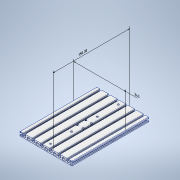
# Autodesk Inventor part: T_20240
Saved by Autodesk Inventor 2021 (Build 250183000, 183)
## iProperties
Created: 2022-05-22
Part Number: T_20240
Material: Aluminio 6061
Document SubType Name: Modeling
Designer: 79449
Density: 2.7 g/cm^3
Appearance: Aluminio - Plano
Author: 79449
Autodesk Inventor part; units mm, degrees
ref_plane "YZ Plane" through (0, 0, 0) normal (1, 0, 0) x (0, 1, 0)
ref_plane "XZ Plane" through (0, 0, 0) normal (0, 1, 0) x (-1, 0, 0)
ref_plane "XY Plane" through (0, 0, 0) normal (0, 0, 1) x (1, 0, 0)
sketch "Boceto1" plane through (0, 0, 0) normal (0, 0, 1) x (1, 0, 0)
  line L0 (-120, 0) -> (120, 0)
  line L1 (-120, 0) -> (-120, 20) construction
  line L2 (-120, 20) -> (120, 20) construction
  line L3 (120, 20) -> (120, 0) construction
  line L4 (-120, 14.15) -> (-117.15, 14.15)
  line L5 (-120, 5.85) -> (-117.15, 5.85)
  line L6 (-117.15, 2.85) -> (-110.15, 2.85)
  line L7 (-117.15, 5.85) -> (-117.15, 2.85)
  line L8 (-117.15, 14.15) -> (-117.15, 17.15)
  line L9 (-117.15, 17.15) -> (-110.15, 17.15)
  line L10 (-120, 5.85) -> (-120, 0)
  line L11 (-120, 14.15) -> (-120, 20)
  line L12 (-120, 20) -> (-104, 20)
  line L13 (-104, 20) -> (-104, 16)
  line L14 (-104, 16) -> (-107, 16)
  line L15 (-107, 16) -> (-107, 8.85)
  line L16 (-107, 8.85) -> (-104, 8.85)
  line L17 (-104, 8.85) -> (-104, 6)
  line L18 (-104, 6) -> (-95.7, 6)
  line L19 (-95.7, 6) -> (-95.7, 8.85)
  line L20 (-95.7, 8.85) -> (-92.7, 8.85)
  line L21 (-92.7, 8.85) -> (-92.7, 16)
  line L22 (-92.7, 16) -> (-95.7, 16)
  line L23 (-95.7, 16) -> (-95.7, 20)
  line L24 (-95.7, 20) -> (-79.9, 20)
  line L25 (-84.05, 14) -> (-75.75, 14)
  line L26 (-79.9, 20) -> (-79.9, 0) construction
  line L27 (-84.05, 14) -> (-84.05, 11.15)
  line L28 (-75.75, 14) -> (-75.75, 11.15)
  line L29 (-84.05, 11.15) -> (-87.05, 11.15)
  line L30 (-75.75, 11.15) -> (-72.75, 11.15)
  line L31 (-72.75, 11.15) -> (-72.75, 4)
  line L32 (-87.05, 11.15) -> (-87.05, 4)
  line L33 (-87.05, 4) -> (-72.75, 4)
  line L34 (-110.15, 17.15) -> (-110.15, 2.85)
  line L35 (-99.85, 6) -> (-99.85, 20) construction
  line L36 (-59.95, 20) -> (-59.95, 0) construction
  line L37 (-39.8, 20) -> (-279.8, 20) construction
  line L38 (-39.8, 20) -> (-55.8, 20)
  line L39 (-55.8, 20) -> (-55.8, 16)
  line L40 (-55.8, 16) -> (-52.8, 16)
  line L41 (-52.8, 16) -> (-52.8, 8.85)
  line L42 (-52.8, 8.85) -> (-55.8, 8.85)
  line L43 (-55.8, 8.85) -> (-55.8, 6)
  line L44 (-55.8, 6) -> (-64.1, 6)
  line L45 (-64.1, 6) -> (-64.1, 8.85)
  line L46 (-64.1, 8.85) -> (-67.1, 8.85)
  line L47 (-67.1, 8.85) -> (-67.1, 16)
  line L48 (-67.1, 16) -> (-64.1, 16)
  line L49 (-64.1, 16) -> (-64.1, 20)
  line L50 (-64.1, 20) -> (-79.9, 20)
  line L51 (-75.75, 14) -> (-84.05, 14)
  line L52 (-75.75, 14) -> (-75.75, 11.15)
  line L53 (-84.05, 14) -> (-84.05, 11.15)
  line L54 (-75.75, 11.15) -> (-72.75, 11.15)
  line L55 (-84.05, 11.15) -> (-87.05, 11.15)
  line L56 (-87.05, 11.15) -> (-87.05, 4)
  line L57 (-72.75, 11.15) -> (-72.75, 4)
  line L58 (-72.75, 4) -> (-87.05, 4)
  line L59 (-59.95, 6) -> (-59.95, 20) construction
  line L60 (-35.85, 14) -> (-44.15, 14)
  line L61 (-40, 20) -> (-40, 0) construction
  line L62 (-35.85, 14) -> (-35.85, 11.15)
  line L63 (-44.15, 14) -> (-44.15, 11.15)
  line L64 (-35.85, 11.15) -> (-32.85, 11.15)
  line L65 (-44.15, 11.15) -> (-47.15, 11.15)
  line L66 (-47.15, 11.15) -> (-47.15, 4)
  line L67 (-32.85, 11.15) -> (-32.85, 4)
  line L68 (-32.85, 4) -> (-47.15, 4)
  line L69 (-35.85, 14) -> (-35.85, 11.15)
  line L70 (-35.85, 11.15) -> (-32.85, 11.15)
  line L71 (-32.85, 11.15) -> (-32.85, 4)
  line L72 (-44.15, 11.15) -> (-47.15, 11.15)
  line L73 (-47.15, 11.15) -> (-47.15, 4)
  line L74 (-44.15, 14) -> (-35.85, 14)
  line L75 (-47.15, 4) -> (-32.85, 4)
  line L76 (-44.15, 14) -> (-44.15, 11.15)
  line L77 (40, 20) -> (-200, 20) construction
  line L78 (-20.05, 20) -> (-20.05, 0) construction
  line L79 (-15.9, 20) -> (-0.1, 20)
  line L80 (-40.2, 20) -> (199.8, 20) construction
  line L81 (-15.9, 8.85) -> (-12.9, 8.85)
  line L82 (-40.2, 20) -> (-24.2, 20)
  line L83 (-27.2, 16) -> (-27.2, 8.85)
  line L84 (-24.2, 8.85) -> (-24.2, 6)
  line L85 (-27.2, 8.85) -> (-24.2, 8.85)
  line L86 (-24.2, 16) -> (-27.2, 16)
  line L87 (-15.9, 6) -> (-15.9, 8.85)
  line L88 (-24.2, 20) -> (-24.2, 16)
  line L89 (-20.05, 6) -> (-20.05, 20) construction
  line L90 (-24.2, 6) -> (-15.9, 6)
  line L91 (-12.9, 8.85) -> (-12.9, 16)
  line L92 (-12.9, 16) -> (-15.9, 16)
  line L93 (-15.9, 16) -> (-15.9, 20)
  line L94 (-4.25, 14) -> (4.05, 14)
  line L95 (4.05, 14) -> (-4.25, 14)
  line L96 (4.05, 14) -> (4.05, 11.15)
  line L97 (4.05, 11.15) -> (7.05, 11.15)
  line L98 (4.05, 14) -> (4.05, 11.15)
  line L99 (-0.1, 20) -> (-0.1, 0) construction
  line L100 (-4.25, 14) -> (-4.25, 11.15)
  line L101 (-4.25, 14) -> (-4.25, 11.15)
  line L102 (-4.25, 11.15) -> (-7.25, 11.15)
  line L103 (7.05, 11.15) -> (7.05, 4)
  line L104 (7.05, 11.15) -> (7.05, 4)
  line L105 (-4.25, 11.15) -> (-7.25, 11.15)
  line L106 (7.05, 4) -> (-7.25, 4)
  line L107 (-7.25, 4) -> (7.05, 4)
  line L108 (4.05, 11.15) -> (7.05, 11.15)
  line L109 (-7.25, 11.15) -> (-7.25, 4)
  line L110 (-7.25, 11.15) -> (-7.25, 4)
  line L111 (119.8, 20) -> (-120.2, 20) construction
  line L112 (40, 20) -> (-200, 20) construction
  line L113 (12.7, 8.85) -> (12.7, 16)
  line L114 (15.7, 8.85) -> (12.7, 8.85)
  line L115 (15.7, 16) -> (15.7, 20)
  line L116 (19.85, 20) -> (19.85, 0) construction
  line L117 (19.85, 6) -> (19.85, 20) construction
  line L118 (24, 20) -> (24, 16)
  line L119 (24, 8.85) -> (24, 6)
  line L120 (24, 6) -> (15.7, 6)
  line L121 (27, 16) -> (27, 8.85)
  line L122 (24, 16) -> (27, 16)
  line L123 (12.7, 16) -> (15.7, 16)
  line L124 (15.7, 20) -> (-0.1, 20)
  line L125 (15.7, 6) -> (15.7, 8.85)
  line L126 (27, 8.85) -> (24, 8.85)
  line L127 (-40.2, 20) -> (199.8, 20) construction
  line L128 (40, 20) -> (24, 20)
  line L129 (39.8, 20) -> (39.8, 0) construction
  line L130 (43.95, 14) -> (35.65, 14)
  line L131 (35.65, 14) -> (43.95, 14)
  line L132 (46.95, 4) -> (32.65, 4)
  line L133 (32.65, 4) -> (46.95, 4)
  line L134 (35.65, 14) -> (35.65, 11.15)
  line L135 (35.65, 14) -> (35.65, 11.15)
  line L136 (35.65, 11.15) -> (32.65, 11.15)
  line L137 (32.65, 11.15) -> (32.65, 4)
  line L138 (35.65, 11.15) -> (32.65, 11.15)
  line L139 (32.65, 11.15) -> (32.65, 4)
  line L140 (43.95, 14) -> (43.95, 11.15)
  line L141 (43.95, 11.15) -> (46.95, 11.15)
  line L142 (43.95, 11.15) -> (46.95, 11.15)
  line L143 (46.95, 11.15) -> (46.95, 4)
  line L144 (46.95, 11.15) -> (46.95, 4)
  line L145 (43.95, 14) -> (43.95, 11.15)
  line L146 (199.6, 20) -> (-40.4, 20) construction
  line L147 (119.8, 20) -> (-120.2, 20) construction
  line L148 (39.6, 20) -> (279.6, 20) construction
  line L149 (-40.2, 20) -> (199.8, 20) construction
  line L150 (39.6, 20) -> (279.6, 20) construction
  line L151 (119.8, 20) -> (-120.2, 20) construction
  line L152 (55.6, 20) -> (55.6, 16)
  line L153 (59.75, 6) -> (59.75, 20) construction
  line L154 (59.75, 20) -> (59.75, 0) construction
  line L155 (55.6, 6) -> (63.9, 6)
  line L156 (63.9, 16) -> (63.9, 20)
  line L157 (63.9, 8.85) -> (66.9, 8.85)
  line L158 (66.9, 16) -> (63.9, 16)
  line L159 (66.9, 8.85) -> (66.9, 16)
  line L160 (63.9, 20) -> (79.7, 20)
  line L161 (55.6, 8.85) -> (55.6, 6)
  line L162 (52.6, 16) -> (52.6, 8.85)
  line L163 (55.6, 16) -> (52.6, 16)
  line L164 (52.6, 8.85) -> (55.6, 8.85)
  line L165 (39.6, 20) -> (55.6, 20)
  line L166 (63.9, 6) -> (63.9, 8.85)
  line L167 (239.5, 20) -> (-0.5, 20) construction
  line L168 (159.7, 20) -> (-80.3, 20) construction
  line L169 (79.5, 20) -> (319.5, 20) construction
  line L170 (-0.3, 20) -> (239.7, 20) construction
  line L171 (79.5, 20) -> (319.5, 20) construction
  line L172 (159.7, 20) -> (-80.3, 20) construction
  line L173 (79.5, 20) -> (95.5, 20)
  line L174 (79.7, 20) -> (79.7, 0) construction
  line L175 (75.55, 14) -> (83.85, 14)
  line L176 (83.85, 14) -> (75.55, 14)
  line L177 (86.85, 11.15) -> (86.85, 4)
  line L178 (86.85, 11.15) -> (86.85, 4)
  line L179 (75.55, 14) -> (75.55, 11.15)
  line L180 (75.55, 14) -> (75.55, 11.15)
  line L181 (86.85, 4) -> (72.55, 4)
  line L182 (72.55, 4) -> (86.85, 4)
  line L183 (72.55, 11.15) -> (72.55, 4)
  line L184 (72.55, 11.15) -> (72.55, 4)
  line L185 (75.55, 11.15) -> (72.55, 11.15)
  line L186 (75.55, 11.15) -> (72.55, 11.15)
  line L187 (83.85, 14) -> (83.85, 11.15)
  line L188 (83.85, 14) -> (83.85, 11.15)
  line L189 (83.85, 11.15) -> (86.85, 11.15)
  line L190 (83.85, 11.15) -> (86.85, 11.15)
  line L191 (159.7, 20) -> (-80.3, 20) construction
  line L192 (-80.1, 20) -> (159.9, 20) construction
  line L193 (79.9, 20) -> (63.9, 20)
  line L194 (-0.3, 20) -> (239.7, 20) construction
  line L195 (-0.3, 20) -> (239.7, 20) construction
  line L196 (79.9, 20) -> (-160.1, 20) construction
  line L197 (239.5, 20) -> (-0.5, 20) construction
  line L198 (159.7, 20) -> (-80.3, 20) construction
  line L199 (79.5, 20) -> (319.5, 20) construction
  line L200 (-0.3, 20) -> (239.7, 20) construction
  line L201 (79.5, 20) -> (319.5, 20) construction
  line L202 (159.7, 20) -> (-80.3, 20) construction
  line L203 (95.5, 20) -> (95.5, 16)
  line L204 (99.65, 6) -> (99.65, 20) construction
  line L205 (99.65, 20) -> (99.65, 0) construction
  line L206 (95.5, 6) -> (103.8, 6)
  line L207 (103.8, 16) -> (103.8, 20)
  line L208 (103.8, 8.85) -> (106.8, 8.85)
  line L209 (106.8, 16) -> (103.8, 16)
  line L210 (106.8, 8.85) -> (106.8, 16)
  line L211 (103.8, 20) -> (119.6, 20)
  line L212 (95.5, 8.85) -> (95.5, 6)
  line L213 (92.5, 16) -> (92.5, 8.85)
  line L214 (95.5, 16) -> (92.5, 16)
  line L215 (92.5, 8.85) -> (95.5, 8.85)
  line L216 (79.5, 20) -> (95.5, 20)
  line L217 (103.8, 6) -> (103.8, 8.85)
  line L218 (159.7, 20) -> (-80.3, 20) construction
  line L219 (-80.1, 20) -> (159.9, 20) construction
  line L220 (-0.3, 20) -> (239.7, 20) construction
  line L221 (-0.3, 20) -> (239.7, 20) construction
  line L222 (119.8, 20) -> (-120.2, 20) construction
  line L223 (119.8, 20) -> (-120.2, 20) construction
  line L224 (119.8, 20) -> (-120.2, 20) construction
  line L225 (-120, 20) -> (120, 20) construction
  line L226 (39.6, 20) -> (279.6, 20) construction
  line L227 (199.6, 20) -> (-40.4, 20) construction
  line L228 (-40.2, 20) -> (199.8, 20) construction
  line L229 (-40.2, 20) -> (199.8, 20) construction
  line L230 (-40.2, 20) -> (199.8, 20) construction
  line L231 (119.8, 0) -> (-120.2, 0)
  line L232 (119.8, 0) -> (119.8, 20) construction
  line L233 (119.8, 20) -> (-120.2, 20) construction
  line L234 (119.8, 14.15) -> (116.95, 14.15)
  line L235 (119.8, 5.85) -> (116.95, 5.85)
  line L236 (116.95, 2.85) -> (109.95, 2.85)
  line L237 (116.95, 5.85) -> (116.95, 2.85)
  line L238 (116.95, 14.15) -> (116.95, 17.15)
  line L239 (116.95, 17.15) -> (109.95, 17.15)
  line L240 (119.8, 5.85) -> (119.8, 0)
  line L241 (119.8, 14.15) -> (119.8, 20)
  line L242 (119.8, 20) -> (103.8, 20)
  line L243 (109.95, 17.15) -> (109.95, 2.85)
  line L244 (39.6, 20) -> (279.6, 20) construction
  line L245 (-40.2, 20) -> (199.8, 20) construction
  line L246 (-120, 20) -> (120, 20) construction
  line L247 (-40.2, 20) -> (199.8, 20) construction
  line L248 (-120, 20) -> (120, 20) construction
  line L249 (-120, 20) -> (120, 20) construction
  line L250 (-80.1, 20) -> (159.9, 20) construction
  line L251 (-120, 20) -> (120, 20) construction
  line L252 (-120, 20) -> (120, 20) construction
  line L253 (-120, 20) -> (120, 20) construction
  line L254 (119.8, 20) -> (-120.2, 20) construction
  point P0 (0, 0)
  point P1 (0, 0)
  point P2 (-79.9, 14)
  point P3 (-40, 14)
  point P4 (-0.1, 14)
  point P5 (39.8, 14)
  point P6 (79.7, 14)
  point P7 (119.8, 0)
  dimension "d0" = 240
  dimension "d1" = 20
  dimension "d2" = 8.3
  dimension "d6" = 7
  dimension "d7" = 2.85
  dimension "d8" = 2.85
  dimension "d9" = 2.85
  dimension "d10" = 3
  dimension "d11" = 3
  dimension "d12" = 7
  dimension "d13" = 16
  dimension "d15" = 4
  dimension "d17" = 14.3
  dimension "d19" = 4
  dimension "d22" = 2.85
  dimension "d23" = 15.8
  dimension "d24" = 6
  dimension "d25" = 6
  dimension "d26" = 8.3
  dimension "d27" = 8.3
  dimension "d29" = 3
  dimension "d30" = 8.3
  dimension "d31" = 2.85
  dimension "d32" = 2.85
  dimension "d33" = 3
  dimension "d34" = 3
  dimension "d35" = 14.3
  dimension "d36" = 7.15
  dimension "d37" = 7.15
  dimension "d38" = 7.15
  dimension "d39" = 19.95
  dimension "d40" = 19.95
  constraints: 510 end point, 270 symmetric about line, 75 point on line, 10 horizontal, 10 perpendicular, 9 vertical, 3 midpoint, 2 collinear, 1 coincident
  measures "d0" distance of L0.start L0.end
  measures "d1" distance of L0.start L1.end
  measures "d2" distance between parallel lines of L5 L4
  measures "d6" distance of L6.start L6.end
  measures "d7" distance between parallel lines of L0 L6
  measures "d8" distance of L4.start L4.end
  measures "d9" distance of L5.start L5.end
  measures "d10" distance of L5.end L6.start
  measures "d11" distance of L4.end L8.end
  measures "d12" distance of L8.end L9.end
  measures "d13" distance of L1.end L12.end
  measures "d15" distance of L12.end L13.end
  measures "d17" distance between parallel lines of L21 L15
  measures "d19" distance of L22.end L23.end
  measures "d22" distance of L18.end L19.end
  measures "d23" distance of L23.end L24.end
  measures "d24" distance between parallel lines of L0 L18
  measures "d25" distance between parallel lines of L25 L24
  measures "d26" distance between parallel lines of L19 L17
  measures "d27" distance between parallel lines of L13 L23
  measures "d29" distance of L19.end L20.end
  measures "d30" distance of L25.start L25.end
  measures "d31" distance of L25.start L27.end
  measures "d32" distance of L25.end L28.end
  measures "d33" distance of L27.end L29.end
  measures "d34" distance of L28.end L30.end
  measures "d35" distance between parallel lines of L32 L31
  measures "d36" distance of L14.end L15.end
  measures "d37" distance of L30.end L31.end
  measures "d38" distance of L29.end L32.end
  measures "d39" distance between parallel lines of L26 L35
  measures "d40" distance between parallel lines of L36 L26
extrude "Extrusión1" add sketch "Boceto1" along normal blind 350
fillet "Empalme1" radius 2 4 edges at (119.8, 20, 175) (119.8, 0, 175) (-120, 20, 175) (-120, 0, 175)
sketch "Boceto2" plane through (-15.9, 20, 0) normal (0, 1, 0) x (1, 0, 0)
  line L0 (15.9, 0) -> (15.9, -350) construction
  circle A0 centre (15.9, -330.27) radius 4
  line L1 (31.6, -350) -> (0, -350) projected
  line L2 (15.9, -175) -> (-107.5519, -175) construction
  line L3 (-56.85, 0) -> (-56.85, -350) projected
  circle A1 centre (15.9, -234.27) radius 4
  circle A2 centre (15.9, -19.73) radius 4
  circle A3 centre (15.9, -115.73) radius 4
  circle A4 centre (28.9, -156) radius 2.1
  circle A5 centre (28.9, -194) radius 2.1
  line L4 (22.95, 0) -> (22.95, -350) projected
  circle A6 centre (2.9, -156) radius 2.1
  circle A7 centre (2.9, -194) radius 2.1
  dimension "d52" = 8
  dimension "d53" = 19.73
  dimension "d54" = 8
  dimension "d55" = 96
  dimension "d58" = 4.2
  dimension "d59" = 19
  dimension "d60" = 19
  dimension "d61" = 4.2
  dimension "d62" = 13
  dimension "d63" = 13
  constraints: 8 centre point, 4 end point, 4 symmetric about line, 3 point on line, 1 midpoint, 1 perpendicular, 1 vertical, 4 other
  measures "d52" diameter of A0
  measures "d53" distance from line of L1 A0.centre
  measures "d54" diameter of A1
  measures "d55" distance of A0.centre A1.centre
  measures "d58" diameter of A4
  measures "d59" distance from line of A4.centre L2
  measures "d60" distance from line of L2 A5.centre
  measures "d61" diameter of A5
  measures "d62" distance from line of L0 A4.centre
  measures "d63" distance from line of L0 A5.centre
extrude "Extrusión2" cut sketch "Boceto2" against normal through all
sketch "Boceto3" plane through (-15.9, 20, 0) normal (0, 1, 0) x (1, 0, 0)
  arc A0 (28.6, -158.0785) -> (28.6, -153.9215) centre (28.9, -156) ccw projected
  circle A1 centre (28.9, -156) radius 4
  line L0 (11.65, 0) -> (11.65, -350) projected
  circle A2 centre (2.9, -156) radius 2.1 projected
  circle A3 centre (2.9, -156) radius 4
  circle A4 centre (2.9, -194) radius 2.1 projected
  circle A5 centre (2.9, -194) radius 4
  circle A6 centre (28.9, -194) radius 2.1 projected
  circle A7 centre (28.9, -194) radius 4
  point P0 (15.9, 0)
  dimension "d64" = 8
  dimension "d65" = 8
  dimension "d67" = 8
  dimension "d68" = 8
  constraints: 4 centre point, 4 coincident
  measures "d64" diameter of A1
  measures "d65" diameter of A3
  measures "d67" diameter of A5
  measures "d68" diameter of A7
extrude "Extrusión3" cut sketch "Boceto3" against normal up to surface (16 mm away)
